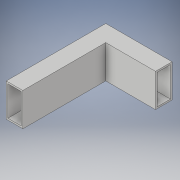
# Autodesk Inventor part: left arm
Saved by Autodesk Inventor 2018 (Build 220112000, 112)
## iProperties
Created: 2019-01-16
Part Number: left arm
Material: Generic
Document SubType Name: Modeling
Designer: s-4008082
Density: 1 g/cm^3
Appearance: Default
Author: s-4008082
Autodesk Inventor part; units mm, degrees
ref_plane "YZ Plane" through (0, 0, 0) normal (1, 0, 0) x (0, 1, 0)
ref_plane "XZ Plane" through (0, 0, 0) normal (0, 1, 0) x (-1, 0, 0)
ref_plane "XY Plane" through (0, 0, 0) normal (0, 0, 1) x (1, 0, 0)
sketch "Sketch15" plane through (0, 0, 0) normal (1, 0, 0) x (0, 1, 0)
  line L0 (0, 0) -> (50.8, 0)
  line L1 (50.8, 0) -> (50.8, 25.4)
  line L2 (50.8, 25.4) -> (0, 25.4)
  line L3 (0, 25.4) -> (0, 0)
  line L4 (48.26, 22.86) -> (2.54, 22.86)
  line L5 (2.54, 22.86) -> (2.54, 2.54)
  line L6 (2.54, 2.54) -> (48.26, 2.54)
  line L7 (48.26, 2.54) -> (48.26, 22.86)
  dimension "d46" = 25.4
  dimension "d47" = 50.8
  dimension "d48" = 2.54
  dimension "d49" = 2.54
  dimension "d50" = 2.54
  dimension "d51" = 2.54
  constraints: 16 end point, 4 parallel, 2 horizontal, 2 perpendicular
  measures "d46" distance of L0.end L1.end
  measures "d47" distance of L1.end L2.end
  measures "d48" distance between parallel lines of L1 L7
  measures "d49" distance between parallel lines of L2 L4
  measures "d50" distance between parallel lines of L3 L5
  measures "d51" distance between parallel lines of L0 L6
extrude "Extrusion12" add sketch "Sketch15" along normal blind 76.2
sketch "Sketch17" plane through (0, 0, 0) normal (0, 0, -1) x (-1, 0, 0)
  line L0 (0, 2.54) -> (-76.2, 2.54) projected
  line L1 (0, 48.26) -> (-76.2, 48.26) projected
  line L2 (-73.617, 2.54) -> (-3.1161, 2.54)
  line L3 (-3.1161, 2.54) -> (-3.1161, 48.26)
  line L4 (-3.1161, 48.26) -> (-73.617, 48.26)
  line L5 (-73.617, 48.26) -> (-73.617, 2.54)
  point P0 (0, 0)
  constraints: 8 end point, 2 parallel, 2 point on line, 1 horizontal, 1 perpendicular
extrude "Extrusion14" add sketch "Sketch17" along normal blind 2.54
sketch "Sketch20" plane through (0, 0, 0) normal (0, 0, -1) x (-1, 0, 0)
  line L0 (0, 0) -> (25.4, 0)
  line L1 (25.4, 0) -> (0, 0)
  line L2 (0, 0) -> (0, 50.8)
  line L3 (0, 50.8) -> (25.4, 50.8)
  line L4 (25.4, 50.8) -> (25.4, 0)
  line L5 (22.86, 48.26) -> (2.54, 48.26)
  line L6 (2.54, 48.26) -> (2.54, 2.54)
  line L7 (2.54, 2.54) -> (22.86, 2.54)
  line L8 (22.86, 2.54) -> (22.86, 48.26)
  line L9 (0, 0) -> (0, 50.8) projected
  dimension "d71" = 25.4
  dimension "d72" = 50.8
  dimension "d73" = 2.54
  dimension "d74" = 2.54
  dimension "d75" = 2.54
  dimension "d76" = 2.54
  dimension "d78" = 0
  constraints: 18 end point, 4 parallel, 2 horizontal, 2 perpendicular
  measures "d71" distance of L2.end L3.end
  measures "d72" distance of L1.end L2.end
  measures "d73" distance between parallel lines of L3 L5
  measures "d74" distance between parallel lines of L2 L6
  measures "d75" distance between parallel lines of L1 L7
  measures "d76" distance between parallel lines of L4 L8
  measures "d78" distance between parallel lines of L9 L2
extrude "Extrusion16" add sketch "Sketch20" against normal blind 152.4
equation "\"d49\" = d48"
equation "\"d50\" = d48"
equation "\"d51\" = d48"
equation "\"d73\" = d77"
equation "\"d74\" = d77"
equation "\"d75\" = d77"
equation "\"d76\" = d77"
equation "\"d77\" = 2.54"
body "Solid2"
